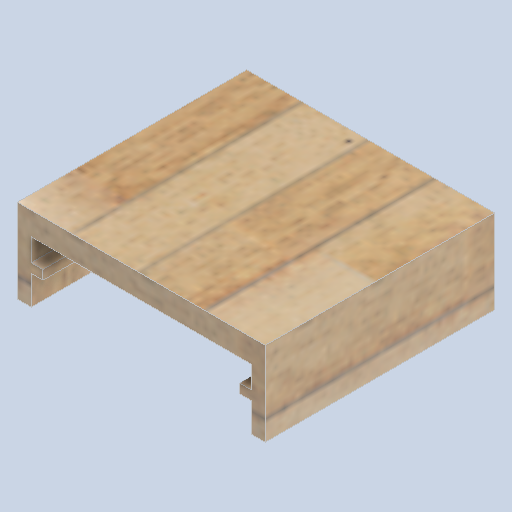
# Autodesk Inventor part: Part8
Saved by Autodesk Inventor 2022 (Build 260153000, 153)
## iProperties
Created: 2022-04-11
Part Number: Part8
Material: Wood (Maple)
Document SubType Name: Modeling
Designer: MacBook
Density: 0.67 g/cm^3
Appearance: Natural Maple - Glossy Dark Tint
Author: MacBook
Autodesk Inventor part; units mm, degrees
ref_plane "YZ Plane" through (0, 0, 0) normal (1, 0, 0) x (0, 1, 0)
ref_plane "XZ Plane" through (0, 0, 0) normal (0, 1, 0) x (-1, 0, 0)
ref_plane "XY Plane" through (0, 0, 0) normal (0, 0, 1) x (1, 0, 0)
sketch "Sketch1" plane through (0, 0, 0) normal (0, 1, 0) x (-1, 0, 0)
  line L0 (-106.3625, -98.425) -> (106.3625, -98.425)
  line L1 (106.3625, -98.425) -> (106.3625, 98.425)
  line L2 (106.3625, 98.425) -> (-106.3625, 98.425)
  line L3 (-106.3625, 98.425) -> (-106.3625, -98.425)
  line L4 (-106.3625, -98.425) -> (106.3625, 98.425) construction
  line L5 (106.3625, -98.425) -> (-106.3625, 98.425) construction
  point P0 (0, 0)
  dimension "d0" = 212.725
  dimension "d1" = 196.85
  constraints: 12 end point, 2 midpoint, 2 parallel, 1 horizontal, 1 perpendicular
  measures "d0" distance between parallel lines of L3 L1
  measures "d1" distance between parallel lines of L0 L2
extrude "Extrusion1" add sketch "Sketch1" against normal blind 72.05
sketch "Sketch2" plane through (-106.3625, 0, 98.425) normal (0, 0, 1) x (1, 0, 0)
  line L0 (0, -72.05) -> (212.725, -72.05) projected
  line L1 (11.906, -20) -> (200.819, -20)
  line L2 (200.819, -20) -> (200.819, -72.05)
  line L3 (200.819, -72.05) -> (11.906, -72.05)
  line L4 (11.906, -72.05) -> (11.906, -20)
  line L5 (0, 0) -> (212.725, 0) projected
  line L6 (0, 0) -> (0, -72.05) projected
  line L7 (212.725, 0) -> (212.725, -72.05) projected
  point P0 (106.3625, 0)
  point P1 (0, -36.025)
  point P2 (212.725, -36.025)
  dimension "d4" = 20
  dimension "d5" = 188.913
  dimension "d6" = 11.906
  dimension "d7" = 11.906
  constraints: 8 end point, 2 midpoint, 2 parallel, 1 horizontal, 1 perpendicular, 1 point on line
  measures "d4" distance between parallel lines of L5 L1
  measures "d5" distance between parallel lines of L2 L4
  measures "d6" distance from line of point (0, -36.025) L4
  measures "d7" distance from line of point (212.725, -36.025) L2
extrude "Extrusion2" cut sketch "Sketch2" against normal blind 172 contours L4 L1 L2 L0
sketch "Sketch3" plane through (-106.3625, 0, 98.425) normal (0, 0, 1) x (1, 0, 0)
  line L0 (11.906, -72.05) -> (11.906, -20) projected
  line L1 (11.906, -39.05) -> (21.906, -39.05)
  line L2 (21.906, -39.05) -> (21.906, -47.05)
  line L3 (21.906, -47.05) -> (11.906, -47.05)
  line L4 (11.906, -47.05) -> (11.906, -39.05)
  line L5 (200.819, -20) -> (200.819, -72.05) projected
  line L6 (200.819, -39.05) -> (190.819, -39.05)
  line L7 (190.819, -39.05) -> (190.819, -47.05)
  line L8 (190.819, -47.05) -> (200.819, -47.05)
  line L9 (200.819, -47.05) -> (200.819, -39.05)
  line L10 (11.906, -20) -> (200.819, -20) projected
  point P0 (106.3625, 0)
  point P1 (16.906, -39.05)
  point P2 (11.906, -47.05)
  dimension "d10" = 10
  dimension "d11" = 10
  dimension "d12" = 19.05
  dimension "d13" = 8
  constraints: 16 end point, 4 parallel, 4 point on line, 2 horizontal, 2 perpendicular, 1 midpoint
  measures "d10" distance between parallel lines of L0 L2
  measures "d11" distance between parallel lines of L5 L7
  measures "d12" distance from line of L10 point (16.906, -39.05)
  measures "d13" distance between parallel lines of L1 L3
extrude "Extrusion3" add sketch "Sketch3" against normal blind 172
sketch "Sketch4" plane through (0, -72.05, 0) normal (0, -1, 0) x (1, 0, 0)
  line L0 (-106.3625, -98.425) -> (106.3625, -98.425) projected
  line L1 (-102.4, -98.425) -> (-65.887, -98.425)
  line L2 (-65.887, -98.425) -> (-65.887, -76.425)
  line L3 (-65.887, -76.425) -> (-102.4, -76.425)
  line L4 (-102.4, -76.425) -> (-102.4, -98.425)
  line L5 (65.887, -98.425) -> (102.4, -98.425)
  line L6 (102.4, -98.425) -> (102.4, -76.425)
  line L7 (102.4, -76.425) -> (65.887, -76.425)
  line L8 (65.887, -76.425) -> (65.887, -98.425)
  line L9 (-106.3625, 98.425) -> (-106.3625, -98.425) projected
  point P0 (0, 0)
  point P1 (102.4, -87.425)
  point P2 (65.887, -87.425)
  dimension "d16" = 36.513
  dimension "d17" = 36.513
  dimension "d18" = 22
  dimension "d19" = 22
  dimension "d20" = 131.774
  dimension "d21" = 3.9625
  constraints: 16 end point, 4 parallel, 2 horizontal, 2 midpoint, 2 perpendicular, 2 point on line
  measures "d16" distance between parallel lines of L2 L4
  measures "d17" distance of point (102.4, -87.425) point (65.887, -87.425)
  measures "d18" distance between parallel lines of L0 L3
  measures "d19" distance between parallel lines of L0 L7
  measures "d20" distance between parallel lines of L8 L2
  measures "d21" distance between parallel lines of L9 L4
extrude "Extrusion4" cut sketch "Sketch4" against normal blind 5
body "Solid1"
